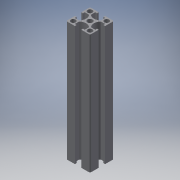
# Autodesk Inventor part: Profile_10
Saved by Autodesk Inventor 2019 (Build 230136000, 136)
## iProperties
Created: 2019-04-07
Part Number: Profile_10
Material: 일반
Document SubType Name: Modeling
Designer: hinmo
Density: 1 g/cm^3
Appearance: 기본값
Author: hinmo
Autodesk Inventor part; units mm, degrees
ref_plane "YZ Plane" through (0, 0, 0) normal (1, 0, 0) x (0, 1, 0)
ref_plane "XZ Plane" through (0, 0, 0) normal (0, 1, 0) x (-1, 0, 0)
ref_plane "XY Plane" through (0, 0, 0) normal (0, 0, 1) x (1, 0, 0)
sketch "스케치1" plane through (0, 0, 0) normal (0, 1, 0) x (-1, 0, 0)
  line L0 (9, 10) -> (-9, 10)
  line L1 (-10, 9) -> (-10, -9)
  line L2 (-9, -10) -> (9, -10)
  line L3 (10, -9) -> (10, 9)
  line L4 (10, 10) -> (-10, -10) construction
  line L5 (-10, 10) -> (10, -10) construction
  line L6 (10, 0) -> (-10, 0)
  line L7 (10, 2.65) -> (10, -2.65)
  line L8 (10, -2.65) -> (8.5, -2.65)
  line L9 (8.5, -2.65) -> (8.5, -4.15)
  line L10 (8.5, -4.15) -> (3.3, -4.15)
  line L11 (3.3, 4.15) -> (8.5, 4.15)
  line L12 (8.5, 4.15) -> (8.5, 2.65)
  line L13 (8.5, 2.65) -> (10, 2.65)
  line L14 (8.5, 4.15) -> (4.9, 4.15)
  line L15 (4.9, 4.15) -> (4.9, -4.15)
  arc A0 (4.9, 4.15) -> (4.9, -4.15) centre (9.482, 0) ccw
  line L16 (4.15, -4.9) -> (-4.15, -4.9)
  line L17 (4.15, -3.3) -> (4.15, -8.5)
  line L18 (4.15, -8.5) -> (2.65, -8.5)
  line L19 (4.15, -8.5) -> (4.15, -4.9)
  line L20 (-2.65, -8.5) -> (-4.15, -8.5)
  line L21 (2.65, -8.5) -> (2.65, -10)
  line L22 (2.65, -10) -> (-2.65, -10)
  line L23 (-2.65, -10) -> (-2.65, -8.5)
  line L24 (-4.15, -8.5) -> (-4.15, -3.3)
  arc A1 (4.15, -4.9) -> (-4.15, -4.9) centre (0, -9.482) ccw
  line L25 (-8.5, 4.15) -> (-3.3, 4.15)
  line L26 (-8.5, 2.65) -> (-8.5, 4.15)
  line L27 (-10, 2.65) -> (-8.5, 2.65)
  line L28 (-10, -2.65) -> (-10, 2.65)
  line L29 (-8.5, -2.65) -> (-10, -2.65)
  line L30 (-4.9, -4.15) -> (-4.9, 4.15)
  arc A2 (-4.9, -4.15) -> (-4.9, 4.15) centre (-9.482, 0) ccw
  line L31 (-8.5, -4.15) -> (-4.9, -4.15)
  line L32 (-8.5, -4.15) -> (-8.5, -2.65)
  line L33 (-3.3, -4.15) -> (-8.5, -4.15)
  line L34 (-4.15, 3.3) -> (-4.15, 8.5)
  line L35 (-4.15, 8.5) -> (-4.15, 4.9)
  line L36 (-4.15, 8.5) -> (-2.65, 8.5)
  line L37 (2.65, 8.5) -> (4.15, 8.5)
  line L38 (-2.65, 8.5) -> (-2.65, 10)
  arc A3 (-4.15, 4.9) -> (4.15, 4.9) centre (0, 9.482) ccw
  line L39 (4.15, 8.5) -> (4.15, 3.3)
  line L40 (-2.65, 10) -> (2.65, 10)
  line L41 (-4.15, 4.9) -> (4.15, 4.9)
  line L42 (2.65, 10) -> (2.65, 8.5)
  line L43 (0, 10) -> (7, 10)
  line L44 (7, 10) -> (7, 7)
  circle A4 centre (7, 7) radius 2
  circle A5 centre (0, 0) radius 2.15
  line L45 (7, 7) -> (-7, 7)
  line L46 (-7, 7) -> (-7, -7)
  line L47 (-7, -7) -> (7, -7)
  circle A6 centre (7, -7) radius 2
  circle A7 centre (-7, -7) radius 2
  circle A8 centre (-7, 7) radius 2
  arc A9 (10, 9) -> (9, 10) centre (9, 9) ccw
  arc A10 (-9, 10) -> (-10, 9) centre (-9, 9) ccw
  arc A11 (-10, -9) -> (-9, -10) centre (-9, -9) ccw
  arc A12 (9, -10) -> (10, -9) centre (9, -9) ccw
  point P0 (0, -10)
  point P1 (-10, 0)
  point P2 (3.3, 4.15)
  point P3 (-3.3, 4.15)
  point P4 (0, 10)
  dimension "d0" = 20
  dimension "d1" = 20
  dimension "d2" = 2.65
  dimension "d3" = 5.3
  dimension "d4" = 1.5
  dimension "d5" = 1.5
  dimension "d6" = 5.2
  dimension "d7" = 8.3
  dimension "d8" = 5.2
  dimension "d9" = 1.5
  dimension "d10" = 3.6
  dimension "d11" = 2.65
  dimension "d12" = 5.3
  dimension "d13" = 1.5
  dimension "d14" = 1.5
  dimension "d15" = 5.2
  dimension "d16" = 8.3
  dimension "d17" = 5.2
  dimension "d18" = 1.5
  dimension "d19" = 3.6
  dimension "d20" = 2.65
  dimension "d21" = 5.3
  dimension "d22" = 1.5
  dimension "d23" = 1.5
  dimension "d24" = 5.2
  dimension "d25" = 8.3
  dimension "d26" = 5.2
  dimension "d27" = 1.5
  dimension "d28" = 3.6
  dimension "d29" = 2.65
  dimension "d30" = 5.3
  dimension "d31" = 1.5
  dimension "d32" = 1.5
  dimension "d33" = 5.2
  dimension "d34" = 8.3
  dimension "d35" = 5.2
  dimension "d36" = 1.5
  dimension "d37" = 3.6
  dimension "d38" = 7
  dimension "d39" = 4
  dimension "d40" = 4.3
  dimension "d41" = 4
  dimension "d42" = 4
  dimension "d43" = 4
  dimension "d44" = 1
  constraints: 96 end point, 24 perpendicular, 23 point on line, 16 point on circle, 13 centre point, 8 tangent, 5 coincident, 4 midpoint, 3 equal radius, 3 horizontal, 2 parallel
  measures "d0" distance of L5.end L4.end
  measures "d1" distance of L4.end L5.start
  measures "d2" distance of L6.start L7.start
  measures "d3" distance of L7.start L7.end
  measures "d4" distance of L7.end L8.end
  measures "d5" distance of L8.end L9.end
  measures "d6" distance of L9.end L10.end
  measures "d7" distance of L10.end L11.start
  measures "d8" distance of L11.start L11.end
  measures "d9" distance of L11.end L12.end
  measures "d10" distance of L11.end L15.start
  measures "d11" distance of point (0, -10) L21.end
  measures "d12" distance of L21.end L22.end
  measures "d13" distance of L22.end L20.start
  measures "d14" distance of L20.start L20.end
  measures "d15" distance of L20.end L24.end
  measures "d16" distance of L24.end L17.start
  measures "d17" distance of L17.start L17.end
  measures "d18" distance of L17.end L21.start
  measures "d19" distance of L17.end L16.start
  measures "d20" distance of point (-10, 0) L28.start
  measures "d21" distance of L28.start L27.start
  measures "d22" distance of L27.start L26.start
  measures "d23" distance of L26.start L26.end
  measures "d24" distance of L26.end L25.end
  measures "d25" distance of L25.end L33.start
  measures "d26" distance of L33.start L33.end
  measures "d27" distance of L33.end L32.end
  measures "d28" distance of L33.end L30.start
  measures "d29" distance of L43.start L38.end
  measures "d30" distance of L38.end L40.end
  measures "d31" distance of L40.end L42.end
  measures "d32" distance of L42.end L37.end
  measures "d33" distance of L37.end L39.end
  measures "d34" distance of L39.end L34.start
  measures "d35" distance of L34.start L36.start
  measures "d36" distance of L36.start L38.start
  measures "d37" distance of L36.start L41.start
  measures "d38" distance of L43.start L43.end
  measures "d39" diameter of A4
  measures "d40" diameter of A5
  measures "d41" diameter of A6
  measures "d42" diameter of A7
  measures "d43" diameter of A8
  measures "d44" radius of A9
extrude "돌출1" add sketch "스케치1" along normal blind 100 contours A9 L3 L13 L12 L11 L39 L45 A4 L44 L0 | L44 A4 L45 L39 L37 L42 L0 | L38 L36 L34 L45 A8 L46 L25 L26 L27 L1 A10 L0 | L3 A12 L2 L21 L18 L17 L10 L9 L8 | L39 L11 A0 L6 A5 A2 L25 L34 A3 | L34 L25 L46 A8 L45 | A0 L10 L17 A1 L24 L33 A2 L6 A5 | L2 A11 L1 L29 L32 L31 L46 A7 L47 L24 L20 L23 | L24 L47 A7 L46 L31 L33
